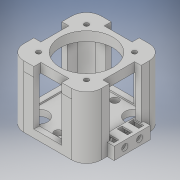
# Autodesk Inventor part: Pillow_Stand
Saved by Autodesk Inventor 2019 (Build 230136000, 136)
## iProperties
Created: 2019-08-16
Part Number: Pillow_Stand
Material: Generic
Document SubType Name: Modeling
Designer: 19879326
Density: 1 g/cm^3
Appearance: Default
Author: 19879326
Autodesk Inventor part; units mm, degrees
ref_plane "YZ Plane" through (0, 0, 0) normal (1, 0, 0) x (0, 1, 0)
ref_plane "XZ Plane" through (0, 0, 0) normal (0, 1, 0) x (-1, 0, 0)
ref_plane "XY Plane" through (0, 0, 0) normal (0, 0, 1) x (1, 0, 0)
sketch "Sketch1" plane through (0, 0, 0) normal (0, 1, 0) x (-1, 0, 0)
  circle A0 centre (0, 0) radius 7.5
  circle A1 centre (0, 18.25) radius 2.5
  circle A2 centre (0, -18.25) radius 2.5
  line L0 (15.5254, 25) -> (-15.5, 25)
  line L1 (-25, 15.5) -> (-25, -15.5)
  line L2 (-15.5, -25) -> (15.5, -25)
  line L3 (25, -15.5) -> (25, 15.5)
  circle A3 centre (15.5, 15.5) radius 6
  circle A4 centre (15.5, -15.5) radius 6
  circle A5 centre (-15.5, -15.5) radius 6
  circle A6 centre (-15.5, 15.5) radius 6
  arc A7 (25, 15.5) -> (15.4745, 25) centre (15.5, 15.5) ccw
  arc A8 (15.5, -25) -> (25, -15.5) centre (15.5, -15.5) ccw
  arc A9 (-25, -15.5) -> (-15.5, -25) centre (-15.5, -15.5) ccw
  arc A10 (-15.5, 25) -> (-25, 15.5) centre (-15.5, 15.5) ccw
  point P0 (25, 0)
  point P1 (0, -25)
  dimension "d0" = 15
  dimension "d1" = 5
  dimension "d2" = 5
  dimension "d3" = 18.25
  dimension "d4" = 18.25
  dimension "d12" = 12
  dimension "d24" = 31
  dimension "d25" = 31
  dimension "d26" = 15.5
  dimension "d27" = 15.5
  dimension "d28" = 15.5
  dimension "d29" = 15.5
  dimension "d30" = 50
  dimension "d31" = 50
  constraints: 11 centre point, 9 point on circle, 8 end point, 5 coincident, 4 tangent, 4 vertical alignment, 3 equal radius, 2 horizontal alignment, 2 midpoint, 2 parallel, 1 horizontal, 1 perpendicular, 1 point on line
  measures "d0" diameter of A0
  measures "d1" diameter of A2
  measures "d2" diameter of A1
  measures "d3" distance of point (0, 0) A1.centre
  measures "d4" distance of point (0, 0) A2.centre
  measures "d12" diameter of A3
  measures "d24" distance of A5.centre A4.centre
  measures "d25" distance of A3.centre A4.centre
  measures "d26" horizontal distance of point (0, 0) A4.centre
  measures "d27" horizontal distance of point (0, 0) A4.centre
  measures "d28" horizontal distance of point (0, 0) A3.centre
  measures "d29" horizontal distance of A6.centre point (0, 0)
  measures "d30" distance between parallel lines of L2 L0
  measures "d31" distance between parallel lines of L1 L3
extrude "Extrusion1" add sketch "Sketch1" along normal blind 4
sketch "Sketch4" plane through (0, 4, 0) normal (0, 1, 0) x (1, 0, 0)
  arc A0 (-15.5, 25) -> (-25, 15.5) centre (-15.5, 15.5) ccw
  arc A1 (25, 15.5) -> (15.5, 25) centre (15.5, 15.5) ccw
  arc A2 (15.5, -25) -> (25, -15.5) centre (15.5, -15.5) ccw
  circle A3 centre (-15.5, -15.5) radius 6 projected
  circle A4 centre (-15.5, 15.5) radius 6 projected
  circle A5 centre (15.5, 15.5) radius 6 projected
  circle A6 centre (15.5, -15.5) radius 6 projected
  line L0 (-15.5254, -25) -> (15.5, -25) projected
  arc A7 (-15.5, 25) -> (-25, 15.5) centre (-15.5, 15.5) ccw projected
  line L1 (15.5, 25) -> (-15.5, 25) projected
  line L2 (25, -15.5) -> (25, 15.5) projected
  arc A8 (15.5, -25) -> (25, -15.5) centre (15.5, -15.5) ccw projected
  line L3 (15.5, -25) -> (-15.5254, -25)
  arc A9 (-25, -15.5) -> (-15.5254, -25) centre (-15.5, -15.5) ccw projected
  line L4 (-25, -15.5) -> (-25, 15.5)
  line L5 (15.5, 25) -> (-15.5, 25) projected
  line L6 (-15.5, 25) -> (15.5, 25)
  line L7 (25, -15.5) -> (25, 15.5) projected
  line L8 (25, -15.5) -> (25, 15.5)
  arc A10 (-25, -15.5) -> (-15.4745, -25) centre (-15.5, -15.5) ccw
  circle A11 centre (-15.5, -15.5) radius 6 projected
  arc A12 (-21.5, -15.5) -> (-15.5, -21.5) centre (-15.5, -15.5) ccw
  arc A13 (-15.5, 21.5) -> (-21.5, 15.4798) centre (-15.5, 15.5) ccw
  arc A14 (21.5, 15.5) -> (15.5, 21.5) centre (15.5, 15.5) ccw
  arc A15 (15.5, -21.5) -> (21.5, -15.5) centre (15.5, -15.5) ccw
  line L9 (-21.5, -15.5) -> (-21.5, 15.5202)
  line L10 (-15.5, 21.5) -> (15.5, 21.5)
  line L11 (21.5, 15.5) -> (21.5, -15.5)
  line L12 (15.5, -21.5) -> (-15.5, -21.5)
  point P0 (0, 0)
  dimension "d32" = 12
  constraints: 17 point on circle, 16 end point, 12 tangent, 8 centre point, 5 coincident, 4 equal radius, 3 collinear, 3 concentric, 2 point on line, 2 vertical, 1 horizontal, 1 parallel, 1 perpendicular
  measures "d32" diameter of A12
extrude "Extrusion2" add sketch "Sketch4" along normal blind 30
sketch "Sketch5" plane through (0, 34, 0) normal (0, 1, 0) x (1, 0, 0)
  circle A0 centre (-15.5, -15.5) radius 1.5
  circle A1 centre (-15.5, 15.5) radius 1.5
  circle A2 centre (15.5, 15.5) radius 1.5
  circle A3 centre (15.5, -15.5) radius 1.5
  arc A4 (-15.5, -21.5) -> (-21.5, -15.5) centre (-15.5, -15.5) ccw projected
  arc A5 (-21.5, 15.4798) -> (-15.5, 21.5) centre (-15.5, 15.5) ccw projected
  arc A6 (15.5, 21.5) -> (21.5, 15.5) centre (15.5, 15.5) ccw projected
  arc A7 (21.5, -15.5) -> (15.5, -21.5) centre (15.5, -15.5) ccw projected
  arc A8 (-25, -15.5) -> (-15.5, -25) centre (-15.5, -15.5) ccw
  arc A9 (-15.5, 25) -> (-25, 15.5) centre (-15.5, 15.5) ccw
  arc A10 (25, 15.5) -> (15.5, 25) centre (15.5, 15.5) ccw
  arc A11 (15.5, -25) -> (25, -15.5) centre (15.5, -15.5) ccw
  line L0 (-25, 15.5) -> (-25, -15.5) projected
  line L1 (15.5, 25) -> (-15.5, 25) projected
  line L2 (25, -15.5) -> (25, 15.5) projected
  line L3 (-15.5, 25) -> (15.5, 25)
  arc A12 (15.5, -25) -> (25, -15.5) centre (15.5, -15.5) ccw projected
  line L4 (-25, -15.5) -> (-25, 15.5)
  line L5 (-15.5, -25) -> (15.5, -25)
  line L6 (25, 15.5) -> (25, -15.5)
  circle A13 centre (0, 0) radius 17
  dimension "d35" = 3
  dimension "d38" = 34
  constraints: 11 tangent, 10 point on circle, 9 centre point, 8 end point, 5 coincident, 4 concentric, 3 equal radius, 1 vertical
  measures "d35" diameter of A0
  measures "d38" diameter of A13
extrude "Extrusion3" add sketch "Sketch5" along normal blind 6
sketch "Sketch6" plane through (0, 40, 0) normal (0, 1, 0) x (1, 0, 0)
  line L0 (29.2297, 9) -> (-29.2297, 9)
  line L1 (-29.2297, 9) -> (-29.2297, -9)
  line L2 (-29.2297, -9) -> (29.2297, -9)
  line L3 (29.2297, -9) -> (29.2297, 9)
  line L4 (9, 29.2297) -> (-9, 29.2297)
  line L5 (-9, 29.2297) -> (-9, -29.2297)
  line L6 (-9, -29.2297) -> (9, -29.2297)
  line L7 (9, -29.2297) -> (9, 29.2297)
  line L8 (12, 9) -> (12, -9)
  point P0 (0, 0)
  point P1 (29.2297, 0)
  point P2 (9, 0)
  point P3 (0, -29.2297)
  point P4 (0, -9)
  dimension "d39" = 18
  dimension "d42" = 3
  constraints: 18 end point, 5 perpendicular, 4 midpoint, 4 parallel, 2 horizontal, 2 horizontal alignment, 2 point on line, 2 vertical alignment
  measures "d39" distance of L2.end L0.start
  measures "d42" distance between parallel lines of L7 L8
extrude "Extrusion4" cut sketch "Sketch6" against normal blind 35 contours L8 L2 L7 L0 | L7 L2 L5 L0 | L0 L5 L4 L7 | L5 L2 L1 L0 | L7 L6 L5 L2
sketch "Sketch7" plane through (25, 0, 15.5) normal (1, 0, 0) x (0, 0, -1)
  circle A0 centre (10.75, 7) radius 1.2
  circle A1 centre (20.25, 7) radius 1.2
  line L0 (0, 0) -> (31, 0) projected
  point P0 (15.5, 0)
  dimension "d43" = 7
  dimension "d44" = 2.4
  dimension "d45" = 9.5
  dimension "d46" = 4.75
  constraints: 2 centre point, 1 equal radius, 1 horizontal alignment
  measures "d43" distance from line of L0 A0.centre
  measures "d44" diameter of A0
  measures "d45" distance of A1.centre A0.centre
  measures "d46" horizontal distance of point (15.5, 0) A1.centre
extrude "Extrusion5" cut sketch "Sketch7" against normal blind 45
sketch "Sketch8" plane through (0, 0, 0) normal (0, -1, 0) x (1, 0, 0)
  line L0 (27.5, 10.2) -> (20.8, 10.2)
  line L1 (20.8, 10.2) -> (20.8, -10.2)
  line L2 (20.8, -10.2) -> (27.5, -10.2)
  line L3 (27.5, -10.2) -> (27.5, 10.2)
  line L4 (25, 15.5) -> (25, -15.5) projected
  point P0 (0, 0)
  point P1 (27.5, 0)
  point P2 (25, 0)
  dimension "d49" = 20.4
  dimension "d50" = 6.7
  dimension "d51" = 2.5
  constraints: 8 end point, 2 midpoint, 2 parallel, 1 horizontal, 1 horizontal alignment, 1 perpendicular
  measures "d49" distance of L2.end L0.start
  measures "d50" distance of L1.end L2.end
  measures "d51" distance between parallel lines of L3 L4
extrude "Extrusion6" cut sketch "Sketch8" against normal blind 10
sketch "Sketch9" plane through (0, 4, 0) normal (0, 1, 0) x (1, 0, 0)
  line L0 (21.5, 10.2) -> (21.5, 15.5) projected
  line L1 (21.5, 10.2) -> (20.8, 10.2)
  line L2 (19.8, 11.2) -> (21.5, 11.2)
  line L3 (21.5, 11.2) -> (21.5, 10.2)
  line L4 (20.8, 10.2) -> (20.8, -10.2)
  line L5 (21.5, -11.2) -> (19.8, -11.2)
  line L6 (19.8, -11.2) -> (19.8, 11.2)
  line L7 (20.8, -10.2) -> (25, -10.2) projected
  line L8 (21.5, -11.2) -> (21.5, -10.2)
  line L9 (21.5, -10.2) -> (20.8, -10.2)
  line L10 (20.8, -10.2) -> (20.8, 10.2) projected
  line L11 (21.5, -10.2) -> (20.8, -10.2) projected
  point P0 (0, 0)
  point P1 (20.8, 0)
  dimension "d54" = 1
  dimension "d55" = 1
  dimension "d56" = 1
  constraints: 16 end point, 4 point on line, 2 midpoint, 2 parallel, 1 horizontal, 1 perpendicular
  measures "d54" distance between parallel lines of L2 L1
  measures "d55" distance between parallel lines of L4 L6
  measures "d56" distance between parallel lines of L7 L5
extrude "Extrusion7" add sketch "Sketch9" along normal blind 3
sketch "Sketch10" plane through (0, 10, 0) normal (0, -1, 0) x (1, 0, 0)
  line L0 (21.5, -10.2) -> (21.5, 10.2) projected
  line L1 (25, -10.2) -> (21.5, -10.2) projected
  line L2 (25, 10.2) -> (25, -10.2) projected
  line L3 (21.5, 10.2) -> (25, 10.2) projected
  line L4 (21.5, 10.2) -> (20.8, 10.2)
  line L5 (20.8, 10.2) -> (20.8, -10.2)
  line L6 (20.8, -10.2) -> (21.5, -10.2)
  line L7 (21.5, -10.2) -> (21.5, 10.2)
  point P0 (0, 0)
  constraints: 8 end point, 2 parallel, 1 horizontal, 1 perpendicular
extrude "Extrusion8" cut sketch "Sketch10" against normal up to next
sketch "Sketch12" plane through (9, 40, 14.4222) normal (-1, 0, 0) x (0, 0, 1)
  line L0 (7.0778, -6) -> (0, -6) projected
  line L1 (0, 0) -> (6, 0)
  line L2 (6, 0) -> (6, -6)
  line L3 (6, -6) -> (0, -6)
  line L4 (0, -6) -> (0, 0)
  line L5 (-28.8444, -6) -> (-35.9222, -6) projected
  line L6 (-39.4222, 0) -> (-28.8444, 0) projected
  line L7 (-28.8444, -6) -> (-34.8444, -6)
  line L8 (-34.8444, -6) -> (-34.8444, 0)
  line L9 (-34.8444, 0) -> (-28.8444, 0)
  line L10 (-28.8444, 0) -> (-28.8444, -6)
  point P0 (-14.4222, -40)
  point P1 (0, 0)
  dimension "d63" = 6
  dimension "d64" = 6
  dimension "d65" = 6
  constraints: 16 end point, 4 parallel, 3 point on line, 2 horizontal, 2 perpendicular
  measures "d63" distance of L2.end L3.end
  measures "d64" distance of L8.end L9.end
  measures "d65" distance of L1.end L2.end
extrude "Extrusion9" add sketch "Sketch12" along normal up to next
sketch "Sketch13" plane through (-25, 40, -9) normal (0, 0, 1) x (1, 0, 0)
  line L0 (10.5778, 0) -> (10.5778, -6) projected
  line L1 (10.5778, 0) -> (4.5778, 0)
  line L2 (4.5778, 0) -> (4.5778, -6)
  line L3 (4.5778, -6) -> (10.5778, -6)
  line L4 (10.5778, -6) -> (10.5778, 0)
  point P0 (25, -40)
  dimension "d68" = 6
  dimension "d69" = 6
  constraints: 8 end point, 2 parallel, 1 horizontal, 1 perpendicular
  measures "d68" distance of L3.end L2.end
  measures "d69" distance of L2.end L1.end
extrude "Extrusion10" add sketch "Sketch13" along normal up to next
sketch "Sketch14" plane through (0, 40, 0) normal (0, 1, 0) x (1, 0, 0)
  circle A0 centre (0, 0) radius 7.5 projected
  circle A1 centre (0, 0) radius 17
  arc A2 (9, -14.4222) -> (9, 14.4222) centre (0, 0) ccw projected
  constraints: 1 centre point, 1 coincident, 1 concentric
extrude "Extrusion11" cut sketch "Sketch14" against normal blind 6
sketch "Sketch15" plane through (0, 0, 0) normal (0, -1, 0) x (1, 0, 0)
  line L0 (20.8, 10.2) -> (20.8, -10.2) projected
  line L1 (20.8, 10.2) -> (27.5, 10.2)
  line L2 (27.5, 10.2) -> (27.5, -10.2)
  line L3 (27.5, -10.2) -> (20.8, -10.2)
  line L4 (20.8, -10.2) -> (20.8, 10.2)
  line L5 (28.5, 11.7) -> (25, 11.7)
  line L6 (25, -11.7) -> (28.5, -11.7)
  line L7 (28.5, -11.7) -> (28.5, 11.7)
  line L8 (25, 15.5) -> (25, 10.2) projected
  line L9 (25, -10.2) -> (25, -15.5) projected
  line L10 (25, 15.5) -> (25, 10.2) projected
  line L11 (25, 11.7) -> (25, 10.2)
  line L12 (25, -10.2) -> (25, -15.5) projected
  line L13 (25, -10.2) -> (25, -11.7)
  point P0 (0, 0)
  dimension "d74" = 6.7
  dimension "d75" = 1.5
  dimension "d76" = 1.5
  dimension "d77" = 20.4
  dimension "d78" = 1
  constraints: 18 end point, 3 parallel, 2 collinear, 2 horizontal, 2 point on line, 1 perpendicular
  measures "d74" distance of L2.end L3.end
  measures "d75" distance between parallel lines of L5 L1
  measures "d76" distance between parallel lines of L6 L3
  measures "d77" distance of L1.end L2.end
  measures "d78" distance between parallel lines of L2 L7
extrude "Extrusion12" add sketch "Sketch15" against normal blind 7 contours L8 L5 L7 L6 L9 L3 L2 L1
sketch "Sketch16" plane through (0, 7, 0) normal (0, 1, 0) x (1, 0, 0)
  line L0 (28.5, 11.7) -> (25, 11.7) projected
  line L1 (28.5, 11.7) -> (25, 11.7)
  line L2 (25, 11.7) -> (25, -11.7)
  line L3 (25, -11.7) -> (28.5, -11.7)
  line L4 (28.5, -11.7) -> (28.5, 11.7)
  line L5 (21.5, 11.2) -> (19.8, 11.2) projected
  line L6 (21.5, 11.2) -> (19.8, 11.2)
  line L7 (19.8, 11.2) -> (19.8, -11.2)
  line L8 (19.8, -11.2) -> (21.5, -11.2)
  line L9 (21.5, -11.2) -> (21.5, 11.2)
  line L10 (20.8, 10.2) -> (21.5, 10.2) projected
  line L11 (25, -11.7) -> (25, -10.2) projected
  line L12 (21.5, 10.2) -> (25, 10.2)
  line L13 (25, 10.2) -> (25, -10.2)
  line L14 (25, -10.2) -> (21.5, -10.2)
  line L15 (21.5, -10.2) -> (21.5, 10.2)
  point P0 (0, 0)
  point P1 (25, 10.2)
  point P2 (27.5, 10.2)
  point P3 (27.5, -10.2)
  point P4 (20.8, -10.2)
  point P5 (27.5, -10.2)
  point P6 (28.5, -11.7)
  point P7 (21.5, -10.2)
  constraints: 24 end point, 6 parallel, 3 horizontal, 3 perpendicular
extrude "Extrusion14" add sketch "Sketch16" along normal blind 1
sketch "Sketch17" plane through (0, 7, 0) normal (0, -1, 0) x (1, 0, 0)
  line L0 (27.5, 10.2) -> (27.5, -10.2) projected
  line L1 (20.8, 10.2) -> (20.8, -10.2) projected
  line L2 (27.5, 9.8) -> (20.8, 9.8)
  line L3 (20.8, 9.8) -> (20.8, 6.6)
  line L4 (20.8, 6.6) -> (27.5, 6.6)
  line L5 (27.5, 6.6) -> (27.5, 9.8)
  line L6 (27.5, -2.2) -> (20.8, -2.2)
  line L7 (20.8, -2.2) -> (20.8, 1)
  line L8 (20.8, 1) -> (27.5, 1)
  line L9 (27.5, 1) -> (27.5, -2.2)
  line L10 (27.5, -9.5) -> (20.8, -9.5)
  line L11 (20.8, -9.5) -> (20.8, -6.3)
  line L12 (20.8, -6.3) -> (27.5, -6.3)
  line L13 (27.5, -6.3) -> (27.5, -9.5)
  line L14 (20.8, 10.2) -> (27.5, 10.2) projected
  point P0 (0, 0)
  point P1 (27.5, 8.2)
  point P2 (27.5, -0.6)
  point P3 (27.5, -7.9)
  dimension "d94" = 2
  dimension "d95" = 8.8
  dimension "d96" = 7.3
  dimension "d97" = 3.2
  dimension "d98" = 3.2
  dimension "d99" = 3.2
  constraints: 24 end point, 6 parallel, 6 point on line, 3 horizontal, 3 midpoint, 3 perpendicular
  measures "d94" distance from line of L14 point (27.5, 8.2)
  measures "d95" distance of point (27.5, -0.6) point (27.5, 8.2)
  measures "d96" distance of point (27.5, -7.9) point (27.5, -0.6)
  measures "d97" distance between parallel lines of L2 L4
  measures "d98" distance between parallel lines of L6 L8
  measures "d99" distance between parallel lines of L10 L12
extrude "Extrusion15" cut sketch "Sketch17" against normal blind 1 contours L0 L4 L1 L2 | L0 L6 L1 L8 | L0 L10 L1 L12
sketch "Sketch18" plane through (28.5, 0, 11.7) normal (1, 0, 0) x (0, 0, -1)
  line L0 (5.1, 7) -> (10.7, 7) projected
  circle A0 centre (6.95, 4) radius 1
  circle A1 centre (16.45, 4) radius 1
  line L1 (1.5, 0) -> (1.5, 7) projected
  point P0 (11.7, 0)
  dimension "d102" = 2
  dimension "d103" = 9.5
  dimension "d104" = 5.45
  dimension "d105" = 3
  constraints: 2 centre point, 1 equal radius, 1 horizontal alignment
  measures "d102" diameter of A0
  measures "d103" distance of A1.centre A0.centre
  measures "d104" distance from line of A0.centre L1
  measures "d105" distance from line of L0 A0.centre
extrude "Extrusion16" cut sketch "Sketch18" against normal blind 12.75
sketch "Sketch19" plane through (28.5, 0, 11.7) normal (1, 0, 0) x (0, 0, -1)
  arc A0 (5.95, 4) -> (7.95, 4) centre (6.95, 4) ccw projected
  circle A1 centre (6.95, 4) radius 2
  circle A2 centre (16.45, 4) radius 1 projected
  circle A3 centre (16.45, 4) radius 2
  circle A4 centre (6.95, 4) radius 1 projected
  circle A5 centre (16.45, 4) radius 1 projected
  line L0 (23.4, 0) -> (0, 0) projected
  line L1 (23.4, 0) -> (23.4, 8) projected
  line L2 (0, 8) -> (23.4, 8) projected
  line L3 (0, 0) -> (0, 8) projected
  point P0 (11.7, 0)
  dimension "d108" = 4
  dimension "d109" = 4
  constraints: 2 centre point, 2 coincident
  measures "d108" diameter of A1
  measures "d109" diameter of A3
extrude "Extrusion17" add sketch "Sketch19" along normal blind 1 contours L0 L3 L2 L1
sketch "Sketch20" plane through (28.5, 4, 4.75) normal (1, 0, 0) x (0, 0, -1)
  circle A0 centre (0, 0) radius 1 projected
  circle A1 centre (0, 0) radius 2 projected
  circle A2 centre (9.5, 0) radius 2 projected
  circle A3 centre (9.5, 0) radius 1 projected
  point P0 (4.75, -4)
extrude "Extrusion18" cut sketch "Sketch20" against normal blind 0.5
body "Solid1"
